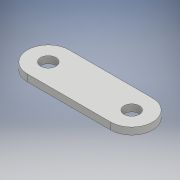
# Autodesk Inventor part: Suporte
Saved by Autodesk Inventor 2018 (Build 220112000, 112)
## iProperties
Created: 2021-08-02
Part Number: Suporte
Material: Generic
Document SubType Name: Modeling
Designer: L08619
Density: 1 g/cm^3
Appearance: Default
Author: L08619
Autodesk Inventor part; units mm, degrees
ref_plane "YZ Plane" through (0, 0, 0) normal (1, 0, 0) x (0, 1, 0)
ref_plane "XZ Plane" through (0, 0, 0) normal (0, 1, 0) x (-1, 0, 0)
ref_plane "XY Plane" through (0, 0, 0) normal (0, 0, 1) x (1, 0, 0)
sketch "Sketch1" plane through (0, 0, 0) normal (0, 0, 1) x (1, 0, 0)
  circle A0 centre (0, 0) radius 11
  arc A1 (0, 30) -> (0, -30) centre (0, 0) ccw
  line L0 (0, 30) -> (120, 30)
  circle A2 centre (120, 0) radius 11
  line L1 (0, -30) -> (120, -30)
  arc A3 (120, -30) -> (120, 30) centre (120, 0) ccw
  dimension "d0" = 22
  dimension "d1" = 30
  dimension "d2" = 120
  dimension "d3" = 22
  dimension "d6" = 120
  constraints: 5 point on circle, 4 centre point, 4 end point, 3 coincident, 2 horizontal, 1 vertical alignment
  measures "d0" diameter of A0
  measures "d1" radius of A1
  measures "d2" distance of L0.start L0.end
  measures "d3" diameter of A2
  measures "d6" distance of L1.start L1.end
extrude "Extrusion1" add sketch "Sketch1" along normal mid plane 10
equation "\"d6\" = d2"
body "Solid1"
